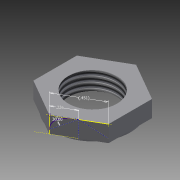
# Autodesk Inventor part: 13_8
Saved by Autodesk Inventor 2015 (Build 190159000, 159)
## iProperties
Created: 2015-04-01
Part Number: 13_8
Material: Generic
Document SubType Name: Modeling
Designer: WASHHSST
Density: 1 g/cm^3
Appearance: Default
Author: WASHHSST
Autodesk Inventor part; units mm, degrees
ref_plane "YZ Plane" through (0, 0, 0) normal (1, 0, 0) x (0, 1, 0)
ref_plane "XZ Plane" through (0, 0, 0) normal (0, 1, 0) x (-1, 0, 0)
ref_plane "XY Plane" through (0, 0, 0) normal (0, 0, 1) x (1, 0, 0)
sketch "Sketch1" plane through (0, 0, 0) normal (0, 1, 0) x (-1, 0, 0)
  circle A0 centre (0, 0) radius 9.9187
  line L0 (9.9187, -5.7266) -> (0, -11.4531)
  line L1 (0, -11.4531) -> (-9.9187, -5.7266)
  line L2 (-9.9187, -5.7266) -> (-9.9187, 5.7266)
  line L3 (-9.9187, 5.7266) -> (0, 11.4531)
  line L4 (0, 11.4531) -> (9.9187, 5.7266)
  line L5 (9.9187, 5.7266) -> (9.9187, -5.7266)
  line L6 (0, 13.376) -> (0, -12.9473) construction
  point P0 (9.9187, 0)
  dimension "d0" = 19.8374
  constraints: 14 end point, 2 coincident, 1 horizontal alignment, 1 midpoint, 1 parallel, 1 vertical, 15 other
extrude "Extrusion1" add sketch "Sketch1" along normal blind 4.3688
sketch "Sketch2" plane through (0, 0, 0) normal (0, -1, 0) x (1, 0, 0)
  circle A0 centre (0, 0) radius 9.9187
  line L0 (0, 11.4531) -> (9.9187, 5.7266) projected
  constraints: 1 centre point, 1 coincident, 1 tangent
extrude "Extrusion2" add sketch "Sketch2" along normal blind 0.4064
sketch "Sketch3" plane through (0, 4.3688, 0) normal (0, 1, 0) x (1, 0, 0)
  point P0 (0, 0)
  point P1 (0, 0)
  constraints: 1 coincident
hole "Hole1" at (0, 4.3688, 0) direction (0, -1, 0) diameter 12.7508 end through all
thread "Thread1" size "9/16-18 UNF" class "2B" standard "ANSI Unified Screw Threads" full length
sketch "Sketch4" plane through (9.9187, 0, 5.7266) normal (0.5, 0, 0.8660254) x (0.8660254, 0, -0.5)
  line L0 (-11.4531, 4.3688) -> (0, 4.3688) projected
  line L1 (-5.7254, 4.3688) -> (-11.4531, 1.0619) construction
  line L2 (-11.4531, 0) -> (-11.4531, 4.3688) projected
  line L3 (-5.7254, 4.3688) -> (-5.7254, 0) construction
  line L4 (-5.7266, 0) -> (-11.4531, 0) construction
  line L5 (-5.7254, 4.3688) -> (0.0023, 1.0619) construction
  line L6 (-5.7254, 4.3688) -> (-11.4531, 4.3688) construction
  line L7 (-11.4531, 4.3688) -> (-11.4531, 1.0619) construction
  line L8 (-5.7266, 0) -> (-14.3164, 0) construction
  spline S0 degree 2 poles (-5.7254, 4.3688) (-11.4531, 4.3688) (-11.4531, 1.0619) knots 1 1 1 2 2 2
  dimension "d14" = 11.4531
  dimension "d15" = 30
  dimension "d16" = 5.7277
  constraints: 6 end point, 3 point on line, 1 coincident, 1 collinear, 1 perpendicular, 1 symmetric about line, 1 vertical, 3 other
  measures "d14" distance of L0.end L0.start
  measures "d15" angle of L0 L1
  measures "d16" distance between parallel lines of L2 L3
body "Solid1"
